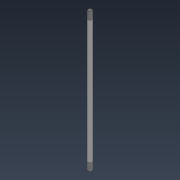
# Autodesk Inventor part: Pret mocujacy
Saved by Autodesk Inventor 2022 (Build 260153000, 153)
## iProperties
Created: 2023-04-12
Part Number: Pret mocujacy
Material: Stainless Steel
Document SubType Name: Modeling
Designer: wikto
Density: 8 g/cm^3
Appearance: Semi-Polished
Author: wikto
Autodesk Inventor part; units mm, degrees
ref_plane "YZ Plane" through (0, 0, 0) normal (1, 0, 0) x (0, 1, 0)
ref_plane "XZ Plane" through (0, 0, 0) normal (0, 1, 0) x (-1, 0, 0)
ref_plane "XY Plane" through (0, 0, 0) normal (0, 0, 1) x (1, 0, 0)
sketch "Sketch1" plane through (0, 0, 0) normal (0, 1, 0) x (-1, 0, 0)
  circle A0 centre (0, 0) radius 4.5
  dimension "d0" = 9
  constraints: 1 centre point, 1 coincident
  measures "d0" diameter of A0
extrude "Extrusion1" add sketch "Sketch1" along normal blind 350
thread "Thread1" size "M9x1.25" class "6g" standard "ISO Metric profile" length 20
thread "Thread2" size "M9x1.25" class "6g" standard "ANSI Metric M Profile" length 20
body "Solid1"
